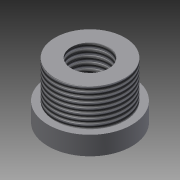
# Autodesk Inventor part: AcmeRoundNut
Saved by Autodesk Inventor 2013 (Build 170138000, 138)
## iProperties
Created: 2012-12-07
Part Number: AcmeRoundNut
Material: Generic
Document SubType Name: Modeling
Designer: istvan.burbank
Density: 1 g/cm^3
Mass: 7.27285 g
Surface Area: 32.9502 cm^2
Volume: 7.27285 cm^3
Author: istvan.burbank
Autodesk Inventor part; units mm, degrees
ref_plane "YZ Plane" through (0, 0, 0) normal (1, 0, 0) x (0, 1, 0)
ref_plane "XZ Plane" through (0, 0, 0) normal (0, 1, 0) x (-1, 0, 0)
ref_plane "XY Plane" through (0, 0, 0) normal (0, 0, 1) x (1, 0, 0)
sketch "Sketch1" plane through (0, 0, 0) normal (0, 1, 0) x (-1, 0, 0)
  circle A0 centre (0, 0) radius 6.35
  circle A1 centre (0, 0) radius 14.224
  dimension "d0" = 12.7
  dimension "d1" = 28.448
  constraints: 2 centre point, 2 coincident
  measures "d0" diameter of A0
  measures "d1" diameter of A1
extrude "Extrusion1" add sketch "Sketch1" along normal blind 19.05
sketch "Sketch2" plane through (0, 19.05, 0) normal (0, 1, 0) x (1, 0, 0)
  circle A0 centre (0, 0) radius 14.224 projected
  circle A1 centre (0, 0) radius 11.8999
  dimension "d6" = 23.7998
  constraints: 1 centre point, 1 coincident
  measures "d6" diameter of A1
extrude "Extrusion2" cut sketch "Sketch2" against normal blind 12.7
thread "Thread3" size "1/2-13 UNC" class "2B" standard "ANSI Unified Screw Threads" length 19.8628
thread "Thread4" size "15/16-16 UN" class "2A" standard "ANSI Unified Screw Threads" length 25.4
body "Solid1"
